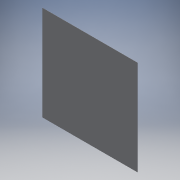
# Autodesk Inventor part: Carpet
Saved by Autodesk Inventor 2018 (Build 220112000, 112)
## iProperties
Created: 2017-09-17
Part Number: Carpet
Material: Generic
Document SubType Name: Modeling
Designer: Techbrick Alt
Density: 1 g/cm^3
Appearance: Default
Author: Techbrick Alt
Autodesk Inventor part; units mm, degrees
ref_plane "YZ Plane" through (0, 0, 0) normal (1, 0, 0) x (0, 1, 0)
ref_plane "XZ Plane" through (0, 0, 0) normal (0, 1, 0) x (-1, 0, 0)
ref_plane "XY Plane" through (0, 0, 0) normal (0, 0, 1) x (1, 0, 0)
sketch "Sketch1" plane through (0, 0, 0) normal (0, 0, 1) x (1, 0, 0)
  line L0 (-1176.6992, 3174.8678) -> (3090.5008, 3174.8678)
  line L1 (3090.5008, 3174.8678) -> (3090.5008, -1092.3322)
  line L2 (3090.5008, -1092.3322) -> (-1176.6992, -1092.3322)
  line L3 (-1176.6992, -1092.3322) -> (-1176.6992, 3174.8678)
  point P0 (0, 0)
  dimension "d0" = 4267.2
  dimension "d1" = 4267.2
  constraints: 8 end point, 2 parallel, 1 horizontal, 1 perpendicular
  measures "d0" distance of L2.end L0.start
  measures "d1" distance of L0.start L0.end
extrude "Carpet" add sketch "Sketch1" along normal blind 6.35
body "Solid1"
